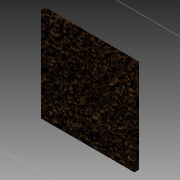
# Autodesk Inventor part: print
Saved by Autodesk Inventor 2015 (Build 190159000, 159)
## iProperties
Created: 2015-12-04
Part Number: print
Material: Generic
Document SubType Name: Modeling
Designer: david
Density: 1 g/cm^3
Appearance: Dirt - Dark Brown
Author: david
Autodesk Inventor part; units mm, degrees
ref_plane "YZ Plane" through (0, 0, 0) normal (1, 0, 0) x (0, 1, 0)
ref_plane "XZ Plane" through (0, 0, 0) normal (0, 1, 0) x (-1, 0, 0)
ref_plane "XY Plane" through (0, 0, 0) normal (0, 0, 1) x (1, 0, 0)
sketch "Sketch1" plane through (0, 0, 0) normal (0, 1, 0) x (-1, 0, 0)
  line L0 (50, -50) -> (-50, -50)
  line L1 (-50, -50) -> (-50, 50)
  line L2 (-50, 50) -> (50, 50)
  line L3 (50, 50) -> (50, -50)
  line L4 (50, -50) -> (-50, 50) construction
  line L5 (-50, -50) -> (50, 50) construction
  point P0 (0, 0)
  dimension "d0" = 100
  dimension "d1" = 100
  constraints: 12 end point, 2 midpoint, 2 parallel, 1 horizontal, 1 perpendicular
  measures "d0" distance of L1.end L2.end
  measures "d1" distance of L0.end L1.end
extrude "Extrusion1" add sketch "Sketch1" along normal blind 5
sketch "Sketch2" plane through (0, 5, 0) normal (0, 1, 0) x (1, 0, 0)
  circle A0 centre (42, 42) radius 4
  circle A1 centre (42, 0) radius 4
  circle A2 centre (42, -42) radius 4
  circle A3 centre (-42, -42) radius 4
  circle A4 centre (-42, 0) radius 4
  circle A5 centre (-42, 42) radius 4
  line L0 (-50, -50) -> (-50, 50) projected
  line L1 (50, 50) -> (-50, 50) projected
  line L2 (-50, -50) -> (50, -50) projected
  line L3 (50, 50) -> (50, -50) projected
  point P0 (0, 0)
  dimension "d4" = 8
  dimension "d5" = 8
  dimension "d6" = 8
  dimension "d7" = 8
  dimension "d8" = 8
  dimension "d9" = 8
  dimension "d10" = 8
  dimension "d11" = 8
  dimension "d12" = 8
  dimension "d13" = 8
  dimension "d14" = 8
  dimension "d15" = 8
  dimension "d16" = 8
  dimension "d17" = 8
  dimension "d18" = 8
  dimension "d19" = 8
  constraints: 6 centre point
  measures "d4" diameter of A0
  measures "d5" diameter of A1
  measures "d6" diameter of A2
  measures "d7" diameter of A3
  measures "d8" diameter of A4
  measures "d9" diameter of A5
  measures "d10" distance from line of L0 A5.centre
  measures "d11" distance from line of L1 A5.centre
  measures "d12" distance from line of L0 A4.centre
  measures "d13" distance from line of L2 A3.centre
  measures "d14" distance from line of L0 A3.centre
  measures "d15" distance from line of L2 A2.centre
  measures "d16" distance from line of L3 A2.centre
  measures "d17" distance from line of L3 A1.centre
  measures "d18" distance from line of A0.centre L1
  measures "d19" distance from line of L3 A0.centre
extrude "Extrusion2" cut sketch "Sketch2" against normal blind 5 contours A0 | A2 | A3 | A5
body "Solid1"
